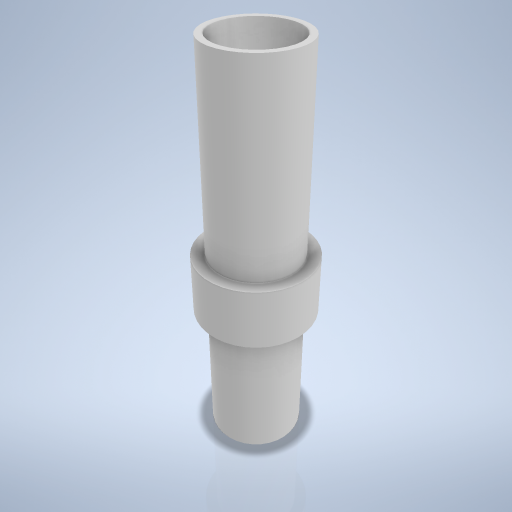
# Autodesk Inventor part: vernindung
Saved by Autodesk Inventor 2024.2 (Build 282272000, 272)
## iProperties
Created: 2024-05-05
Part Number: vernindung
Material: Generisch
Document SubType Name: Modeling
Designer: Fabri
Density: 1 g/cm^3
Appearance: Vorgabe
Author: Fabri
Autodesk Inventor part; units mm, degrees
ref_plane "YZ Plane" through (0, 0, 0) normal (1, 0, 0) x (0, 1, 0)
ref_plane "XZ Plane" through (0, 0, 0) normal (0, 1, 0) x (-1, 0, 0)
ref_plane "XY Plane" through (0, 0, 0) normal (0, 0, 1) x (1, 0, 0)
sketch "Skizze1" plane through (0, 0, 0) normal (0, 1, 0) x (-1, 0, 0)
  line L0 (10.5, 52.028) -> (10.5, 7.028)
  line L1 (10.5, 7.028) -> (13.5, 7.028)
  line L2 (13.5, 7.028) -> (13.5, -7.028)
  line L3 (13.5, -7.028) -> (10.5, -7.028)
  line L4 (10.5, -7.028) -> (10.5, -40.028)
  line L5 (10.5, -40.028) -> (0, -40.028)
  line L6 (0, 52.028) -> (0, -40.028)
  line L7 (0, 0) -> (13.5, 0) construction
  line L8 (10.5, 52.028) -> (0, 52.028)
  point P0 (12, 7.028)
  dimension "d0" = 14.056
  dimension "d1" = 21
  dimension "d2" = 27
  dimension "d14" = 45
  dimension "d15" = 33
  constraints: 18 end point, 4 perpendicular, 2 horizontal, 2 midpoint, 2 point on line, 1 horizontal alignment, 1 vertical
  measures "d0" distance between parallel lines of L3 L1
  measures "d1" diameter of L0 L6
  measures "d2" diameter of L2 L6
  measures "d14" distance between parallel lines of L1 L8
  measures "d15" distance between parallel lines of L5 L3
revolve "Umdrehung1" add sketch "Skizze1" angle 360 about axis through (0, 0, 52.028) along (0, 0, -1)
sketch "Skizze2" plane through (0, 0, 52.028) normal (0, 0, 1) x (1, 0, 0)
  point P0 (0, 0)
  point P1 (0, 0)
  constraints: 1 coincident
hole "Bohrung1" at (0, 0, 52.028) direction (0, 0, -1) diameter 18 end through all
